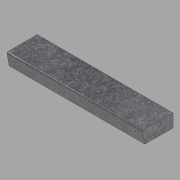
# Autodesk Inventor part: B
Saved by Autodesk Inventor 2022.1 (Build 261234020, 234B)
## iProperties
Created: 2021-12-14
Part Number: B
Material: Granite, Cut, Polished
Document SubType Name: Modeling
Designer: awelt
Density: 2.7 g/cm^3
Appearance: Kasota SN sapphire
Author: awelt
Autodesk Inventor part; units mm, degrees
ref_plane "YZ Plane" through (0, 0, 0) normal (1, 0, 0) x (0, 1, 0)
ref_plane "XZ Plane" through (0, 0, 0) normal (0, 1, 0) x (-1, 0, 0)
ref_plane "XY Plane" through (0, 0, 0) normal (0, 0, 1) x (1, 0, 0)
sketch "Sketch2" plane through (0, 0, 0) normal (1, 0, 0) x (0, 1, 0)
  line L0 (0, 0) -> (0, 152.4)
  line L1 (0, 152.4) -> (342.9, 152.4)
  line L2 (0, 0) -> (330.2, 0)
  line L3 (330.2, 0) -> (355.3918, 137.4098)
  arc A0 (355.3918, 137.4098) -> (342.9, 152.4) centre (342.9, 139.7) ccw
  point P0 (358.14, 152.4)
  dimension "d2" = 152.4
  dimension "d3" = 330.2
  dimension "d4" = 12.7
  dimension "d7" = 342.9
  constraints: 8 end point, 2 point on circle, 2 point on line, 2 tangent, 1 centre point, 1 horizontal, 1 perpendicular, 1 vertical
  measures "d2" distance of L0.start L0.end
  measures "d3" distance of L0.start L2.end
  measures "d4" radius of A0
  measures "d7" distance of L0.end L1.end
extrude "Extrusion1" add sketch "Sketch2" along normal blind 1595.12
body "Solid1"
